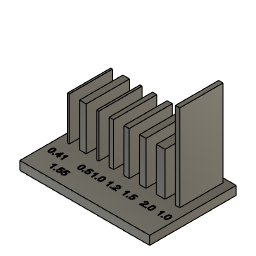
Wall Thickness v19 (Autodesk Fusion 360 design; units mm, degrees)
Autodesk Fusion 360 part; units mm, degrees
sketch "Base" plane through (0, 0, 0) normal (0, 0, 1) x (1, 0, 0)
  line L0 (0, 0) -> (30, 0)
  line L1 (30, 0) -> (30, 20)
  line L2 (30, 20) -> (0, 20)
  line L3 (0, 20) -> (0, 0)
  dimension "d1" = 30
  dimension "d2" = 20
  constraint horizontal L0
  constraint vertical L1
  constraint horizontal L2
  constraint vertical L3
  constraint coincident L0.start L3.end
  measures "d1" distance of L0.start L0.end
  measures "d2" distance of L0.start L2.end
extrude "Extrude1" add sketch "Base" along normal blind 2 makes body 1
sketch "Walls" plane through (0, 0, 2) normal (0, 0, 1) x (-1, 0, 0)
  line L0 (0, -20) -> (0, 0)
  line L1 (0, 0) -> (-30, 0)
  line L2 (-30, 0) -> (-30, -20)
  line L3 (-30, -20) -> (0, -20)
  line L4 (0, -20) -> (0, -19) construction
  line L5 (0, -19) -> (-2, -19) construction
  line L6 (-2, -19) -> (-2.41, -19)
  line L7 (-2.41, -19) -> (-4.81, -19) construction
  line L8 (-4.81, -19) -> (-6.36, -19)
  line L9 (-6.36, -19) -> (-8.76, -19) construction
  line L10 (-8.76, -19) -> (-9.26, -19)
  line L11 (-9.26, -19) -> (-11.66, -19) construction
  line L12 (-11.66, -19) -> (-12.66, -19)
  line L13 (-12.66, -19) -> (-15.06, -19) construction
  line L14 (-15.06, -19) -> (-16.26, -19)
  line L15 (-16.26, -19) -> (-18.66, -19) construction
  line L16 (-18.66, -19) -> (-20.16, -19)
  line L17 (-2, -19) -> (-2, -9)
  line L18 (-2.41, -19) -> (-2.41, -9)
  line L19 (-2, -9) -> (-2.41, -9)
  line L20 (-4.81, -19) -> (-4.81, -9)
  line L21 (-4.81, -9) -> (-6.36, -9)
  line L22 (-6.36, -9) -> (-6.36, -19)
  line L23 (-8.76, -19) -> (-8.76, -9)
  line L24 (-8.76, -9) -> (-9.26, -9)
  line L25 (-9.26, -9) -> (-9.26, -19)
  line L26 (-11.66, -19) -> (-11.66, -9)
  line L27 (-11.66, -9) -> (-12.66, -9)
  line L28 (-12.66, -9) -> (-12.66, -19)
  line L29 (-15.06, -19) -> (-15.06, -9)
  line L30 (-15.06, -9) -> (-16.26, -9)
  line L31 (-16.26, -9) -> (-16.26, -19)
  line L32 (-18.66, -19) -> (-18.66, -9)
  line L33 (-18.66, -9) -> (-20.16, -9)
  line L34 (-20.16, -9) -> (-20.16, -19)
  line L35 (-20.16, -19) -> (-22.56, -19) construction
  line L36 (-22.56, -19) -> (-24.56, -19)
  line L37 (-24.56, -19) -> (-26.96, -19) construction
  line L38 (-26.96, -19) -> (-27.96, -19)
  line L39 (-22.56, -19) -> (-22.56, -9)
  line L40 (-22.56, -9) -> (-24.56, -9)
  line L41 (-24.56, -9) -> (-24.56, -19)
  line L42 (-26.96, -19) -> (-26.96, -9)
  line L43 (-26.96, -9) -> (-27.96, -9)
  line L44 (-27.96, -9) -> (-27.96, -19)
  dimension "d5" = 1
  dimension "d6" = 2
  dimension "d7" = 0.41
  dimension "d8" = 2.4
  dimension "d9" = 1.55
  dimension "d11" = 0.5
  dimension "d13" = 1
  dimension "d15" = 1.2
  dimension "d17" = 1.5
  dimension "d18" = 10
  dimension "d49" = 2
  dimension "d50" = 1
  constraint coincident L0.start L3.end
  constraint perpendicular L3 L4
  constraint perpendicular L4 L5
  constraint perpendicular L4 L6
  constraint parallel L6 L7
  constraint parallel L7 L8
  constraint parallel L8 L9
  constraint parallel L9 L10
  constraint parallel L10 L11
  constraint parallel L11 L12
  constraint parallel L12 L13
  constraint parallel L13 L14
  constraint parallel L3 L15
  constraint parallel L15 L16
  constraint perpendicular L5 L17
  constraint perpendicular L7 L18
  constraint perpendicular L18 L19
  constraint perpendicular L8 L20
  constraint perpendicular L20 L21
  constraint perpendicular L8 L22
  constraint perpendicular L10 L23
  constraint perpendicular L23 L24
  constraint perpendicular L10 L25
  constraint perpendicular L12 L26
  constraint perpendicular L26 L27
  constraint perpendicular L13 L28
  constraint perpendicular L14 L29
  constraint perpendicular L29 L30
  constraint perpendicular L15 L31
  constraint perpendicular L15 L32
  constraint perpendicular L32 L33
  constraint perpendicular L16 L34
  constraint equal L18 L20
  constraint equal L20 L23
  constraint equal L18 L26
  constraint equal L18 L29
  constraint equal L18 L32
  constraint equal L7 L9
  constraint equal L7 L11
  constraint equal L7 L13
  constraint equal L7 L15
  constraint perpendicular L34 L35
  constraint perpendicular L34 L36
  constraint parallel L36 L37
  constraint parallel L37 L38
  constraint equal L7 L37
  constraint perpendicular L36 L39
  constraint equal L17 L39
  constraint perpendicular L39 L40
  constraint equal L36 L40
  constraint equal L7 L35
  constraint perpendicular L38 L42
  constraint perpendicular L2 L43
  constraint equal L38 L43
  constraint equal L18 L42
  measures "d5" distance of L0.start L4.end
  measures "d6" distance of L4.end L5.end
  measures "d7" distance of L5.end L6.end
  measures "d8" distance of L6.end L7.end
  measures "d9" distance of L7.end L8.end
  measures "d11" distance of L9.end L10.end
  measures "d13" distance of L11.end L12.end
  measures "d15" distance of L13.end L14.end
  measures "d17" distance of L15.end L16.end
  measures "d18" distance of L5.end L17.end
  measures "d49" distance of L35.end L36.end
  measures "d50" distance of L37.end L38.end
extrude "Extrude2" add sketch "Walls" along normal blind 10 separate body contours L6 L17 L18 L19 | L8 L20 L21 L22 | L10 L23 L24 L25 | L12 L26 L27 L28 | L14 L29 L30 L31 | L16 L32 L33 L34 | L36 L39 L40 L41 makes body 2 at (9.26, 12.3333, 5.3333) makes body 3 at (20.16, 12.3333, 5.3333) makes body 4 at (6.36, 12.3333, 5.3333) makes body 5 at (12.66, 12.3333, 5.3333) makes body 6 at (16.26, 12.3333, 5.3333) makes body 7 at (2, 15.6667, 5.3333) makes body 8 at (22.56, 15.6667, 5.3333)
sketch "Annotate" plane through (0, 0, 2) normal (0, 0, 1) x (-1, 0, 0)
  line L0 (0, -20) -> (0, 0)
  line L1 (0, 0) -> (-30, 0)
  line L2 (-30, 0) -> (-30, -20)
  line L3 (-30, -20) -> (0, -20)
  line L4 (-4.585, -2) -> (-6.585, -2) construction
  line L5 (-6.585, -2) -> (-6.585, -4) construction
  line L6 (-6.585, -4) -> (-4.585, -4) construction
  line L7 (-4.585, -4) -> (-4.585, -2) construction
  line L8 (-1.205, -5) -> (-3.205, -5) construction
  line L9 (-3.205, -5) -> (-3.205, -7) construction
  line L10 (-3.205, -7) -> (-1.205, -7) construction
  line L11 (-1.205, -7) -> (-1.205, -5) construction
  line L12 (-8.01, -5) -> (-10.01, -5) construction
  line L13 (-10.01, -5) -> (-10.01, -7) construction
  line L14 (-10.01, -7) -> (-8.01, -7) construction
  line L15 (-8.01, -7) -> (-8.01, -5) construction
  line L16 (-11.16, -5) -> (-13.16, -5) construction
  line L17 (-13.16, -5) -> (-13.16, -7) construction
  line L18 (-13.16, -7) -> (-11.16, -7) construction
  line L19 (-11.16, -7) -> (-11.16, -5) construction
  line L20 (-14.66, -5) -> (-16.66, -5) construction
  line L21 (-16.66, -5) -> (-16.66, -7) construction
  line L22 (-16.66, -7) -> (-14.66, -7) construction
  line L23 (-14.66, -7) -> (-14.66, -5) construction
  line L24 (-18.41, -5) -> (-20.41, -5) construction
  line L25 (-20.41, -5) -> (-20.41, -7) construction
  line L26 (-20.41, -7) -> (-18.41, -7) construction
  line L27 (-18.41, -7) -> (-18.41, -5) construction
  line L28 (-22.56, -5) -> (-24.56, -5) construction
  line L29 (-24.56, -5) -> (-24.56, -7) construction
  line L30 (-24.56, -7) -> (-22.56, -7) construction
  line L31 (-22.56, -7) -> (-22.56, -5) construction
  line L32 (-26.46, -5) -> (-28.46, -5) construction
  line L33 (-28.46, -5) -> (-28.46, -7) construction
  line L34 (-28.46, -7) -> (-26.46, -7) construction
  line L35 (-26.46, -7) -> (-26.46, -5) construction
  line L36 (-2.205, -9) -> (-2.205, -7) construction
  line L37 (-2, -9) -> (-2.41, -9)
  line L38 (-5.585, -9) -> (-5.585, -4) construction
  line L39 (-4.81, -9) -> (-6.36, -9)
  line L40 (-9.01, -9) -> (-9.01, -7) construction
  line L41 (-8.76, -9) -> (-9.26, -9)
  line L42 (-11.66, -9) -> (-12.66, -9) construction
  line L43 (-12.16, -9) -> (-12.16, -7) construction
  line L44 (-15.66, -9) -> (-15.66, -7) construction
  line L45 (-15.06, -9) -> (-16.26, -9) construction
  line L46 (-19.41, -9) -> (-19.41, -7) construction
  line L47 (-18.66, -9) -> (-20.16, -9) construction
  line L48 (-23.56, -9) -> (-23.56, -7) construction
  line L49 (-22.56, -9) -> (-24.56, -9) construction
  line L50 (-26.96, -9) -> (-27.96, -9)
  line L51 (-27.46, -7) -> (-27.46, -9)
  point P0 (-26.96, -9)
  dimension "d52" = 2
  dimension "d55" = 2
  dimension "d58" = 5
  dimension "d65" = 2
  text T0 "1.55" font "Arial" height 2 align ink ink in box 0 x 0 at (-4.585, -2) x (-1, 0) y (0, -1) spacing 1 kerned height is em
  text T1 "0.41" font "Arial" height 2 align ink ink in box 0 x 0 at (-1.205, -5) x (-1, 0) y (0, -1) spacing 1 kerned height is em
  text T2 "0.5" font "Arial" height 2 align ink ink in box 0 x 0 at (-8.01, -5) x (-1, 0) y (0, -1) spacing 1 kerned height is em
  text T3 "1.0" font "Arial" height 2 align ink ink in box 0 x 0 at (-11.16, -5) x (-1, 0) y (0, -1) spacing 1 kerned height is em
  text T4 "1.2" font "Arial" height 2 align ink ink in box 0 x 0 at (-14.66, -5) x (-1, 0) y (0, -1) spacing 1 kerned height is em
  text T5 "1.5" font "Arial" height 2 align ink ink in box 0 x 0 at (-18.41, -5) x (-1, 0) y (0, -1) spacing 1 kerned height is em
  text T6 "2.0" font "Arial" height 2 align ink ink in box 0 x 0 at (-22.56, -5) x (-1, 0) y (0, -1) spacing 1 kerned height is em
  text T7 "1.0" font "Arial" height 2 align ink ink in box 0 x 0 at (-26.46, -5) x (-1, 0) y (0, -1) spacing 1 kerned height is em
  constraint perpendicular L4 L5
  constraint parallel L4 L6
  constraint parallel L5 L7
  constraint perpendicular L8 L9
  constraint parallel L8 L10
  constraint parallel L9 L11
  constraint perpendicular L12 L13
  constraint parallel L12 L14
  constraint parallel L13 L15
  constraint perpendicular L16 L17
  constraint parallel L16 L18
  constraint parallel L17 L19
  constraint perpendicular L20 L21
  constraint parallel L20 L22
  constraint parallel L21 L23
  constraint perpendicular L24 L25
  constraint parallel L24 L26
  constraint parallel L25 L27
  constraint perpendicular L28 L29
  constraint parallel L28 L30
  constraint parallel L29 L31
  constraint perpendicular L32 L33
  constraint parallel L32 L34
  constraint parallel L33 L35
  constraint equal L7 L35
  constraint equal L7 L31
  constraint equal L7 L15
  constraint equal L7 L19
  constraint equal L7 L11
  constraint equal L7 L27
  constraint equal L7 L23
  constraint parallel L1 L4
  constraint parallel L4 L32
  constraint parallel L4 L28
  constraint parallel L4 L12
  constraint parallel L4 L16
  constraint parallel L4 L8
  constraint parallel L4 L24
  constraint parallel L4 L20
  constraint equal L6 L10
  constraint equal L10 L26
  constraint equal L22 L26
  constraint equal L18 L22
  constraint equal L14 L18
  constraint equal L14 L30
  constraint equal L30 L34
  constraint vertical L36
  constraint midpoint L36.start L37
  constraint midpoint L10 L36.end
  constraint vertical L38
  constraint midpoint L38.start L39
  constraint midpoint L6 L38.end
  constraint vertical L40
  constraint midpoint L40.start L41
  constraint midpoint L14 L40.end
  constraint equal L36 L40
  constraint vertical L43
  constraint midpoint L42 L43.start
  constraint midpoint L18 L43.end
  constraint equal L40 L44
  constraint midpoint L44.start L45
  constraint midpoint L22 L44.end
  constraint perpendicular L44 L45
  constraint parallel L21 L46
  constraint midpoint L46.start L47
  constraint midpoint L26 L46.end
  constraint equal L43 L46
  constraint vertical L48
  constraint midpoint L48.start L49
  constraint midpoint L30 L48.end
  constraint equal L44 L48
  constraint equal L40 L43
  constraint midpoint L34 L51.start
  constraint perpendicular L50 L51
  constraint midpoint L50 L51.end
  constraint equal L48 L51
  measures "d52" distance of L4.start L6.end
  measures "d55" distance of L36.start L36.end
  measures "d58" distance of L38.start L38.end
  measures "d65" distance of L12.start L12.end
extrude "Extrude4" cut sketch "Annotate" against normal blind 0.5 text T1 T0 T2 T3 T4 T5 T6 T7 bodies 1
extrude "Extrude5" add sketch "Walls" along normal blind 20 contours L38 L42 L43 L44 bodies 1
equation "d1 = basel"
equation "d2 = basew"
equation "d5 = fgapw - 2 mm"
equation "d6 = fgapl"
equation "d8 = gap"
equation "d18 = wall"
equation "d20 = wallh"
equation "basew = 20 mm"
equation "basel = 30 mm"
equation "baseh = 2 mm"
equation "gap = 2.4 mm"
equation "fgapw = 3 mm"
equation "fgapl = 2 mm"
equation "wall = 10 mm"
equation "wallh = 10 mm"
equation "texth = 2 mm"
equation "d52 = texth"
equation "textl = 2 mm"
equation "d55 = textgaps"
equation "textgaps = 2 mm"
equation "textgapl = textgaps * 2.5"
equation "d58 = textgapl"
equation "d59 = textcut"
equation "textcut = -0.5 mm"
equation "d65 = textl"
equation "d66 = wallh * 2"
named bodies: "base", "0.5 thick", "1.5 thick", "0.1 thick", "1.0 thick", "1.2 thick", "0.05 thick", "2.0 thick"
